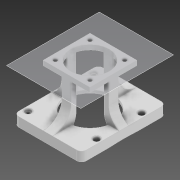
# Autodesk Inventor part: Vacuum BLDC
Saved by Autodesk Inventor 2020 (Build 240168000, 168)
## iProperties
Created: 2022-08-12
Part Number: Vacuum BLDC
Material: Generic
Document SubType Name: Modeling
Designer: Umair
Density: 1 g/cm^3
Appearance: Default
Author: Umair
Autodesk Inventor part; units mm, degrees
ref_plane "YZ Plane" through (0, 0, 0) normal (1, 0, 0) x (0, 1, 0)
ref_plane "XZ Plane" through (0, 0, 0) normal (0, 1, 0) x (-1, 0, 0)
ref_plane "XY Plane" through (0, 0, 0) normal (0, 0, 1) x (1, 0, 0)
sketch "Sketch1" plane through (0, 0, 0) normal (0, 1, 0) x (-1, 0, 0)
  line L0 (0, 0) -> (31, 0)
  line L1 (31, 0) -> (-31, 0)
  line L2 (-31, 0) -> (-31, -24)
  line L3 (-31, -24) -> (-31, 24)
  line L4 (31, 0) -> (31, -35)
  line L5 (31, -35) -> (31, 35)
  line L6 (31, 35) -> (36, 35)
  line L7 (31, -35) -> (36, -35)
  line L8 (36, 35) -> (36, 45)
  line L9 (36, 45) -> (-36, 45)
  line L10 (-36, 45) -> (-36, -34)
  line L11 (36, 45) -> (36, -34)
  line L12 (31, -24) -> (31, -34)
  line L13 (-31, 24) -> (-31, -24)
  line L14 (36, 45) -> (36, -45)
  line L15 (36, -45) -> (-36, -45)
  line L16 (-36, -45) -> (-36, -34)
  circle A0 centre (31, 35) radius 2
  circle A1 centre (31, -35) radius 2
  circle A2 centre (-31, -24) radius 2
  circle A3 centre (-31, 24) radius 2
  dimension "d0" = 31
  dimension "d1" = 62
  dimension "d2" = 24
  dimension "d3" = 48
  dimension "d4" = 35
  dimension "d5" = 70
  dimension "d6" = 5
  dimension "d7" = 5
  dimension "d8" = 10
  dimension "d9" = 72
  dimension "d10" = 79
  dimension "d11" = 90
  dimension "d12" = 4
  dimension "d13" = 4
  dimension "d14" = 4
  dimension "d15" = 4
  constraints: 34 end point, 6 point on line, 4 centre point, 4 coincident, 4 perpendicular, 3 horizontal, 2 vertical, 1 collinear
  measures "d0" distance of L0.start L0.end
  measures "d1" distance of L0.end L1.end
  measures "d2" distance of L1.end L2.end
  measures "d3" distance of L2.end L3.end
  measures "d4" distance of L0.end L4.end
  measures "d5" distance of L4.end L5.end
  measures "d6" distance of L5.end L6.end
  measures "d7" distance of L4.end L7.end
  measures "d8" distance of L6.end L8.end
  measures "d9" distance of L8.end L9.end
  measures "d10" distance of L9.end L10.end
  measures "d11" distance of L8.end L14.end
  measures "d12" diameter of A0
  measures "d13" diameter of A1
  measures "d14" diameter of A2
  measures "d15" diameter of A3
extrude "Extrusion1" add sketch "Sketch1" along normal blind 10 contours L5 A0 L6 L11 L14 L7 A1 L4 | L4 A1 L7 L14 L15 L16 L10 L9 L8 L6 A0 L5
sketch "Sketch2" plane through (0, 10, 0) normal (0, 1, 0) x (1, 0, 0)
  circle A0 centre (0, 0) radius 25
  dimension "d18" = 50
  constraints: 1 centre point, 1 coincident
  measures "d18" diameter of A0
extrude "Extrusion2" cut sketch "Sketch2" against normal blind 10
ref_plane "Work Plane1" through (0, 55, 0) normal (0, 1, 0) x (1, 0, 0)
sketch "Sketch3" plane through (0, 55, 0) normal (0, 1, 0) x (1, 0, 0)
  line L0 (-18.5, -18.5) -> (18.5, -18.5)
  line L1 (18.5, -18.5) -> (18.5, 18.5)
  line L2 (18.5, 18.5) -> (-18.5, 18.5)
  line L3 (-18.5, 18.5) -> (-18.5, -18.5)
  line L4 (-18.5, -18.5) -> (18.5, 18.5) construction
  line L5 (18.5, -18.5) -> (-18.5, 18.5) construction
  circle A0 centre (-18.5, -18.5) radius 2
  circle A1 centre (-18.5, 18.5) radius 2
  circle A2 centre (18.5, 18.5) radius 2
  circle A3 centre (18.5, -18.5) radius 2
  line L6 (25, -25) -> (-25, -25)
  line L7 (-25, -25) -> (-25, 25)
  line L8 (-25, 25) -> (25, 25)
  line L9 (25, 25) -> (25, -25)
  line L10 (25, -25) -> (-25, 25) construction
  line L11 (-25, -25) -> (25, 25) construction
  circle A4 centre (0, 0) radius 20.5
  dimension "d22" = 37
  dimension "d23" = 37
  dimension "d24" = 4
  dimension "d25" = 4
  dimension "d26" = 4
  dimension "d27" = 4
  dimension "d28" = 50
  dimension "d29" = 50
  constraints: 24 end point, 5 centre point, 4 coincident, 4 midpoint, 4 parallel, 2 horizontal, 2 perpendicular
  measures "d22" distance of L2.end L1.end
  measures "d23" distance of L1.end L0.end
  measures "d24" diameter of A0
  measures "d25" diameter of A1
  measures "d26" diameter of A2
  measures "d27" diameter of A3
  measures "d28" distance of L7.end L8.end
  measures "d29" distance of L6.end L7.end
extrude "Extrusion3" add sketch "Sketch3" against normal blind 5 contours A0 L3 A4 L0 | A4 L1 A3 L0 | L3 A1 L2 A4 | A4 L2 A2 L1 | L6 L7 L8 L9
sketch "Sketch4" plane through (0, 50, 0) normal (0, -1, 0) x (1, 0, 0)
  line L0 (-25, 25) -> (25, 25) projected
  line L1 (0, 25) -> (-24.8713, 25)
  line L2 (-24.8713, 25) -> (-15.8713, 25)
  line L3 (0, 25) -> (0, 20.5)
  circle A0 centre (0, 0) radius 20.5 projected
  line L4 (0, 25) -> (-15.8713, 25)
  line L5 (-4.9139, 19.9024) -> (-4.9139, 25)
  line L6 (5.0956, 25) -> (5.0956, 19.8566)
  line L7 (-4.9139, 25) -> (5.0956, 25)
  arc A1 (5.0956, 19.8566) -> (-4.9139, 19.9024) centre (0, 0) ccw
  dimension "d32" = 9
  constraints: 14 end point, 7 point on circle, 3 point on line, 2 perpendicular, 1 centre point, 1 horizontal, 1 midpoint, 1 parallel
  measures "d32" distance of L1.end L2.end
extrude "Extrusion4" add sketch "Sketch4" along normal up to surface (50 mm away) contours L0 L3 A0 L5 | L0 L6 A0 L3
fillet "Fillet2" radius 20 1 edges at (0.0908, 10, 25)
pattern_circular "Circular Pattern1" count 4 over 360 about axis through (0, -10, 0) along (0, 1, 0) of "Extrusion4"
fillet "Fillet3" radius 20 3 edges at (-0.0908, 10, -25) (-25, 10, 0.0908) (25, 10, -0.0908)
fillet "Fillet4" radius 20 3 edges at (-20.4998, 0, 0.0937) (-0.0937, 0, -20.4998) (20.4998, 0, -0.0937)
sketch "Sketch5" plane through (0, 0, 0) normal (0, -1, 0) x (1, 0, 0)
  circle A0 centre (31, 24) radius 2 projected
  circle A1 centre (31, 24) radius 3.25
  circle A2 centre (31.053, -23.9828) radius 3.25
  circle A3 centre (-31, 35) radius 2 projected
  circle A4 centre (-31, 35) radius 3.25
  circle A5 centre (-31, -35) radius 2 projected
  circle A6 centre (-31, -35) radius 3.25
  point P0 (0, 0)
  dimension "d42" = 6.5
  dimension "d43" = 6.5
  dimension "d44" = 6.5
  dimension "d45" = 6.5
  constraints: 4 centre point, 3 coincident
  measures "d42" diameter of A1
  measures "d43" diameter of A2
  measures "d44" diameter of A4
  measures "d45" diameter of A6
extrude "Extrusion5" cut sketch "Sketch5" against normal blind 5 contours A3 | A4 | A5 | A6
sketch "Sketch6" plane through (0, 10, 0) normal (0, 1, 0) x (1, 0, 0)
  arc A0 (32.9488, 23.5505) -> (31.053, 25.9993) centre (31, 24) ccw projected
  circle A1 centre (31, 24) radius 3
  arc A2 (31.053, -25.9993) -> (32.9488, -23.5505) centre (31, -24) ccw projected
  circle A3 centre (31, -24) radius 3
  circle A4 centre (-31, 35) radius 2 projected
  circle A5 centre (-31, 35) radius 3
  circle A6 centre (-31, -35) radius 2 projected
  circle A7 centre (-31, -35) radius 3
  point P0 (0, 0)
  dimension "d48" = 6
  dimension "d49" = 6
  dimension "d50" = 6
  dimension "d51" = 6
  constraints: 4 centre point, 4 coincident
  measures "d48" diameter of A1
  measures "d49" diameter of A3
  measures "d50" diameter of A5
  measures "d51" diameter of A7
extrude "Extrusion6" cut sketch "Sketch6" against normal blind 2 contours A4 | A5 | A6 | A7
extrude "Extrusion7" cut sketch "Sketch6" against normal blind 7 contours A1 | A3
fillet "Fillet5" radius 1 6 edges at (28, 10, -24) (-34, 10, -35) (-34, 10, 35) (28, 10, 24) (-34.25, 0, 35) (-34.25, 0, -35)
fillet "Fillet6" radius 5 4 edges at (-36, 5, -45) (36, 5, -45) (36, 5, 45) (-36, 5, 45)
body "Solid1"
